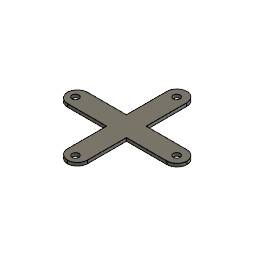
Drone240LX (Autodesk Fusion 360 design; units mm, degrees)
Autodesk Fusion 360 part; units mm, degrees
sketch "Sketch1" plane through (0, 0, 0) normal (0, 1, 0) x (1, 0, 0)
  line L0 (0.4, 76.2) -> (0, 76.2)
  line L1 (12.7, 63.5) -> (12.7, -61.1)
  line L2 (0, -73.8) -> (0.4, -73.8)
  line L3 (-12.3, -61.1) -> (-12.3, 63.5)
  line L4 (-61.1, 12.7) -> (63.5, 12.7)
  line L5 (76.2, 0) -> (76.2, 0.4)
  line L6 (63.5, -12.3) -> (-61.1, -12.3)
  line L7 (-73.8, 0.4) -> (-73.8, 0)
  circle A0 centre (-63.5, 0) radius 4.225
  circle A1 centre (0, 63.5) radius 4.225
  circle A2 centre (63.5, 0) radius 4.225
  circle A3 centre (0, -63.5) radius 4.225
  arc A4 (-73.8, 0.4) -> (-61.1, -12.3) centre (-61.1, 0.4) ccw
  arc A5 (-61.1, 12.7) -> (-73.8, 0) centre (-61.1, 0) ccw
  arc A6 (0.4, 76.2) -> (-12.3, 63.5) centre (0.4, 63.5) ccw
  arc A7 (12.7, 63.5) -> (0, 76.2) centre (0, 63.5) ccw
  arc A8 (76.2, 0) -> (63.5, 12.7) centre (63.5, 0) ccw
  arc A9 (63.5, -12.3) -> (76.2, 0.4) centre (63.5, 0.4) ccw
  arc A10 (-12.3, -61.1) -> (0.4, -73.8) centre (0.4, -61.1) ccw
  arc A11 (0, -73.8) -> (12.7, -61.1) centre (0, -61.1) ccw
  point P0 (-12.3, 76.2)
  point P1 (12.7, 76.2)
  point P2 (-12.3, -73.8)
  point P3 (-73.8, 12.7)
  point P4 (76.2, 12.7)
  point P5 (-73.8, -12.3)
  dimension "d3" = 25
  dimension "d4" = 150
  dimension "d5" = 150
  dimension "d6" = 25
  dimension "d7" = 8.45
  dimension "d8" = 8.45
  dimension "d9" = 8.45
  dimension "d10" = 8.45
  dimension "d11" = 12.7
  constraint horizontal L0
  constraint vertical L1
  constraint horizontal L2
  constraint vertical L3
  constraint horizontal L4
  constraint vertical L5
  constraint horizontal L6
  constraint vertical L7
  constraint coincident P5 L6
  constraint coincident P5 L7
  constraint tangent L6 A4
  constraint tangent L7 A4
  constraint coincident P3 L4
  constraint coincident P3 L7
  constraint tangent L4 A5
  constraint tangent L7 A5
  constraint equal A4 A5
  constraint coincident P0 L0
  constraint coincident P0 L3
  constraint tangent L0 A6
  constraint tangent L3 A6
  constraint equal A4 A6
  constraint coincident P1 L0
  constraint coincident P1 L1
  constraint tangent L0 A7
  constraint tangent L1 A7
  constraint equal A4 A7
  constraint coincident P4 L4
  constraint coincident P4 L5
  constraint tangent L4 A8
  constraint tangent L5 A8
  constraint equal A4 A8
  constraint tangent L5 A9
  constraint tangent L6 A9
  constraint equal A4 A9
  constraint coincident P2 L2
  constraint coincident P2 L3
  constraint tangent L2 A10
  constraint tangent L3 A10
  constraint equal A4 A10
  constraint tangent L1 A11
  constraint tangent L2 A11
  constraint equal A4 A11
  measures "d3" distance of P0 P1
  measures "d4" distance of P0 P2
  measures "d5" distance of P3 P4
  measures "d6" distance of P3 P5
  measures "d7" diameter of A0
  measures "d8" diameter of A1
  measures "d9" diameter of A2
  measures "d10" diameter of A3
  measures "d11" radius of A4
extrude "Extrude1" add sketch "Sketch1" along normal blind 4
